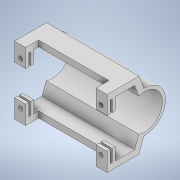
# Autodesk Inventor part: obejmadrążka
Saved by Autodesk Inventor 2022 (Build 260153000, 153)
## iProperties
Created: 2022-04-29
Part Number: obejmadrążka
Material: Ogólny
Document SubType Name: Modeling
Designer: Karle
Density: 1 g/cm^3
Appearance: Domyślna
Author: Karle
Autodesk Inventor part; units mm, degrees
ref_plane "YZ Plane" through (0, 0, 0) normal (1, 0, 0) x (0, 1, 0)
ref_plane "XZ Plane" through (0, 0, 0) normal (0, 1, 0) x (-1, 0, 0)
ref_plane "XY Plane" through (0, 0, 0) normal (0, 0, 1) x (1, 0, 0)
sketch "Szkic1" plane through (0, 0, 0) normal (1, 0, 0) x (0, 1, 0)
  arc A0 (-13.3906, 4.8738) -> (13.3906, 4.8738) centre (0, 0) ccw
  arc A1 (-16.7323, 0.7692) -> (16.7323, 0.7692) centre (0, 0) ccw
  line L0 (13.3906, 4.8738) -> (15.7399, 5.7288)
  line L1 (0, 0) -> (16.75, 0) construction
  line L2 (0, 0) -> (0, 14)
  line L3 (-13.3906, 4.8738) -> (-15.7399, 5.7288)
  line L4 (0, 14) -> (0, 16.75)
  line L5 (12.5, 24) -> (22.5, 24)
  line L6 (-12.5, 24) -> (-22.5, 24)
  line L7 (22.2845, 26.5) -> (12.5, 26.5)
  line L8 (12.5, 26.5) -> (12.5, 24)
  line L9 (22.2845, 26.5) -> (22.2845, 28)
  line L10 (22.2845, 28) -> (12.5, 28)
  line L11 (12.5, 28) -> (12.5, 30.5)
  line L12 (12.5, 30.5) -> (22.2845, 30.5)
  line L13 (-22.5, 24) -> (-12.5, 24)
  line L14 (-12.5, 24) -> (-12.5, 26.5)
  line L15 (-12.5, 26.5) -> (-22.5, 26.5)
  line L16 (-22.5, 26.5) -> (-22.5, 28)
  line L17 (-22.5, 28) -> (-12.5, 28)
  line L18 (-12.5, 28) -> (-12.5, 30.5)
  line L19 (-12.5, 30.5) -> (-22.5, 30.5)
  line L20 (22.5, 24) -> (22.5, 8.1893)
  line L21 (22.5, 8.1893) -> (15.7399, 5.7288)
  line L22 (-22.5, 24) -> (-22.5, 8.1893)
  line L23 (-22.5, 8.1893) -> (-15.7399, 5.7288)
  line L24 (-22.5, 30.5) -> (-27.5, 30.5)
  line L25 (-27.5, 30.5) -> (-27.5, 10.0092)
  line L26 (22.2845, 30.5) -> (27.2845, 30.5)
  line L27 (27.2845, 30.5) -> (27.2845, 10.0135)
  line L28 (20.83, 2.2606) -> (27.2845, 4.6099)
  line L29 (27.2845, 4.6099) -> (27.2845, 10.0135)
  line L30 (20.83, 2.2606) -> (16.7323, 0.7692)
  line L31 (-20.83, 2.2606) -> (-16.7323, 0.7692)
  line L32 (-20.83, 2.2606) -> (-27.5, 4.6099)
  line L33 (-27.5, 4.6099) -> (-27.5, 10.0092)
  dimension "d26" = 5
  dimension "d27" = 5
  constraints: 68 end point, 10 perpendicular, 7 point on line, 6 point on circle, 6 vertical, 4 horizontal, 2 centre point, 2 coincident, 2 parallel
  measures "d26" distance of L19.end L24.end
  measures "d27" distance of L12.end L26.end
extrude "Wyciągnięcie proste1" add sketch "Szkic1" along normal blind 75
sketch "Szkic2" plane through (0, 12.5, 30.5) normal (0, 0, 1) x (1, 0, 0)
  line L0 (0, 14.7845) -> (75, 14.7845) projected
  line L1 (0, 14.7845) -> (9, 14.7845)
  line L2 (75, -40) -> (75, -33.33) projected
  line L3 (75, -40) -> (66, -40)
  line L4 (9, 14.7845) -> (66, 14.7845)
  line L5 (66, 14.7845) -> (66, -40)
  line L6 (66, -40) -> (9, -40)
  line L7 (9, -40) -> (9, 14.7845)
  point P0 (0, -12.5)
  dimension "d32" = 9
  dimension "d33" = 9
  constraints: 12 end point, 2 horizontal, 2 parallel, 1 perpendicular, 1 point on line
  measures "d32" distance of L0.start L1.end
  measures "d33" distance of L2.start L3.end
extrude "Wyciągnięcie proste2" cut sketch "Szkic2" against normal blind 10.5
sketch "Szkic3" plane through (0, 12.5, 30.5) normal (0, 0, 1) x (1, 0, 0)
  line L0 (0, 0) -> (0, 9.7845) projected
  line L1 (5, 0) -> (0, 0)
  circle A0 centre (5, 5) radius 1.75
  line L2 (0, -25) -> (9, -25) projected
  line L3 (5, -25) -> (0, -25)
  circle A1 centre (5, -30) radius 1.75
  line L4 (66, -25) -> (75, -25) projected
  circle A2 centre (70, -30) radius 1.75
  circle A3 centre (70.1447, 5) radius 1.75
  point P0 (0, -12.5)
  dimension "d39" = 3.5
  dimension "d42" = 3.5
  dimension "d46" = 3.5
  dimension "d48" = 3.5
  constraints: 4 centre point, 4 end point, 1 collinear, 1 point on line
  measures "d39" diameter of A0
  measures "d42" diameter of A1
  measures "d46" diameter of A2
  measures "d48" diameter of A3
extrude "Wyciągnięcie proste3" cut sketch "Szkic3" against normal blind 10.5
